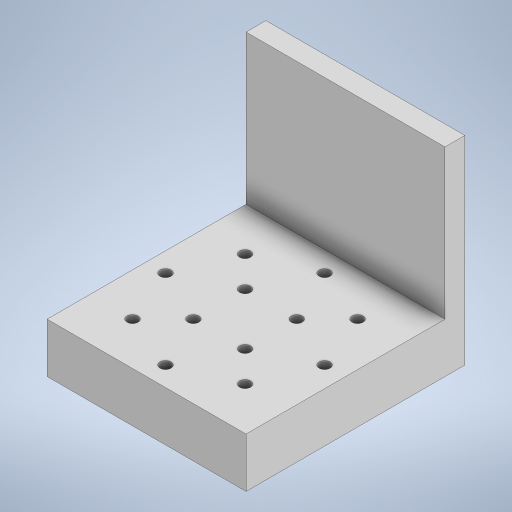
# Autodesk Inventor part: uchwyt chwytak
Saved by Autodesk Inventor 2024 (Build 280153000, 153)
## iProperties
Created: 2025-05-22
Part Number: uchwyt chwytak
Material: Ogólny
Document SubType Name: Modeling
Designer: Paweł
Density: 1 g/cm^3
Appearance: Domyślna
Author: Paweł
Autodesk Inventor part; units mm, degrees
ref_plane "YZ Plane" through (0, 0, 0) normal (1, 0, 0) x (0, 1, 0)
ref_plane "XZ Plane" through (0, 0, 0) normal (0, 1, 0) x (-1, 0, 0)
ref_plane "XY Plane" through (0, 0, 0) normal (0, 0, 1) x (1, 0, 0)
sketch "Szkic1" plane through (0, 0, 0) normal (0, 0, 1) x (1, 0, 0)
  line L0 (-50, 50) -> (50, 50)
  line L1 (50, 50) -> (50, -50)
  line L2 (50, -50) -> (-50, -50)
  line L3 (-50, -50) -> (-50, 50)
  point P0 (0, 0)
  point P1 (0, 50)
  point P2 (-50, 0)
  dimension "d0" = 100
  dimension "d1" = 100
  constraints: 8 end point, 2 midpoint, 2 parallel, 1 horizontal, 1 horizontal alignment, 1 perpendicular, 1 vertical alignment
  measures "d0" distance of L0.start L0.end
  measures "d1" distance of L0.end L1.end
extrude "Wyciągnięcie proste1" add sketch "Szkic1" along normal blind 10
sketch "Szkic2" plane through (0, 0, 10) normal (0, 0, 1) x (1, 0, 0)
  line L0 (-50, -50) -> (50, -50) projected
  line L1 (50, -50) -> (50, 50) projected
  line L2 (-50, -50) -> (50, -50)
  line L3 (50, -50) -> (50, -25)
  line L4 (50, -25) -> (-50, -25)
  line L5 (-50, -25) -> (-50, -50)
  point P0 (0, 0)
  dimension "d4" = 25
  constraints: 8 end point, 2 parallel, 1 horizontal, 1 perpendicular, 1 point on line
  measures "d4" distance between parallel lines of L0 L4
extrude "Wyciągnięcie proste2" add sketch "Szkic2" along normal blind 100
sketch "Szkic3" plane through (-50, -25, 10) normal (0, 1, 0) x (1, 0, 0)
  circle A0 centre (49.7287, -50.229) radius 50
  circle A1 centre (36.7287, -37.229) radius 2.75
  circle A2 centre (36.7287, -63.229) radius 2.75
  circle A3 centre (62.7287, -37.229) radius 2.75
  circle A4 centre (62.7287, -63.229) radius 2.75
  circle A5 centre (78.013, -78.5133) radius 2.75
  circle A6 centre (89.7287, -50.229) radius 2.75
  circle A7 centre (78.013, -21.9447) radius 2.75
  circle A8 centre (49.7287, -10.229) radius 2.75
  circle A9 centre (21.4444, -21.9447) radius 2.75
  circle A10 centre (9.7287, -50.229) radius 2.75
  circle A11 centre (21.4444, -78.5133) radius 2.75
  circle A12 centre (49.7287, -90.229) radius 2.75
  point P0 (50, 10)
  constraints: 13 centre point
extrude "Wyciągnięcie proste3" cut sketch "Szkic3" against normal blind 100 contours A1 | A2 | A3 | A4 | A5 | A6 | A7 | A8 | A9 | A10 | A11 | A12
